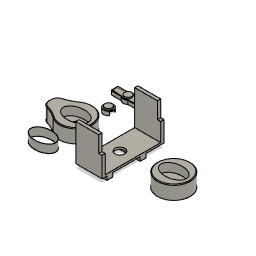
FPLock_Mach (Autodesk Fusion 360 design; units mm, degrees)
Autodesk Fusion 360 part; units mm, degrees
sketch "草图5" plane through (0, 0, 0) normal (0, 1, 0) x (1, 0, 0)
  line L0 (100, -50) -> (140, -50)
  line L1 (140, -50) -> (140, 45)
  line L2 (140, 45) -> (100, 45)
  line L3 (100, 45) -> (100, -50)
  constraint horizontal L0
  constraint vertical L1
  constraint horizontal L2
  constraint vertical L3
extrude "拉伸7" add sketch "草图5" along normal blind 3 makes body 1
sketch "草图6" plane through (0, 3, 0) normal (0, 1, 0) x (-1, 0, 0)
  line L0 (-100, -45) -> (-100, 50)
  line L1 (-100, 50) -> (-140, 50)
  line L2 (-140, 50) -> (-140, -45)
  line L3 (-140, -45) -> (-100, -45)
  line L4 (-100, -40) -> (-140, -40)
  line L5 (-140, -40) -> (-140, -45)
  line L6 (-140, -45) -> (-100, -45)
  line L7 (-100, -45) -> (-100, -40)
  line L8 (-140, 45) -> (-100, 45)
  line L9 (-100, 45) -> (-100, 50)
  line L10 (-100, 50) -> (-140, 50)
  line L11 (-140, 50) -> (-140, 45)
  constraint horizontal L4
  constraint vertical L5
  constraint horizontal L6
  constraint vertical L7
  constraint coincident L2.end L3.start
  constraint coincident L0 L4.start
  constraint horizontal L8
  constraint vertical L9
  constraint horizontal L10
  constraint vertical L11
  constraint coincident L0.end L1.start
  constraint coincident L2 L8.start
extrude "拉伸8" add sketch "草图6" along normal blind 47 contours L0 L2 L3 L4 L5 L6 L7 | L0 L1 L2 L8 L9 L10 L11 bodies 1
sketch "草图7" plane through (0, 3, 0) normal (0, 1, 0) x (-1, 0, 0)
  line L0 (-100, 45) -> (-140, 45)
  line L1 (-140, 45) -> (-140, -40)
  line L2 (-140, -40) -> (-100, -40)
  line L3 (-100, -40) -> (-100, 45)
  circle A0 centre (-120, 2.5) radius 7.5
  dimension "d80" = 15
  measures "d80" diameter of A0
extrude "拉伸9" cut sketch "草图7" against normal blind 3 contours A0 bodies 1
sketch "草图8" plane through (0, 0, -45) normal (0, 0, -1) x (-1, 0, 0)
  line L0 (-140, 0) -> (-100, 0)
  line L1 (-100, 0) -> (-100, 50)
  line L2 (-100, 50) -> (-140, 50)
  line L3 (-140, 50) -> (-140, 0)
sketch "草图11" plane through (0, 0, -45) normal (0, 0, -1) x (-1, 0, 0)
  line L0 (-135, 50) -> (-150, 50)
  line L1 (-150, 50) -> (-150, 25)
  line L2 (-150, 25) -> (-135, 25)
  line L3 (-135, 25) -> (-135, 50)
  constraint horizontal L0
  constraint vertical L1
  constraint horizontal L2
  constraint vertical L3
extrude "拉伸12" cut sketch "草图11" against normal blind 5 bodies 1
sketch "草图12" plane through (0, 0, 50) normal (0, 0, 1) x (1, 0, 0)
  line L0 (100, 0) -> (140, 0)
  line L1 (140, 0) -> (140, 50)
  line L2 (140, 50) -> (100, 50)
  line L3 (100, 50) -> (100, 0)
  line L4 (135, 25) -> (140, 25)
  line L5 (140, 25) -> (140, 50)
  line L6 (140, 50) -> (135, 50)
  line L7 (135, 50) -> (135, 25)
  constraint horizontal L4
  constraint vertical L5
  constraint horizontal L6
  constraint vertical L7
  constraint coincident L1.end L2.start
extrude "拉伸15" cut sketch "草图12" against normal blind 5 contours L1 L2 L4 L5 L6 L7 bodies 1
extrude "拉伸25" cut 2 faces at (138.3333, 25, -43.3333) (136.6667, 25, 48.3333) along direction (0, -1, 0) blind 1 on bodies 1 bodies 1
sketch "草图24" plane through (0, 0, 0) normal (0, -1, 0) x (1, 0, 0)
  circle A0 centre (120, 2.5) radius 7.5
  line L0 (100, 50) -> (100, -45)
  line L1 (100, -45) -> (140, -45)
  line L2 (140, -45) -> (140, 50)
  line L3 (140, 50) -> (100, 50)
  line L4 (140, 2.5) -> (100, 2.5)
  line L5 (120, 2.5) -> (120, -7.5)
  line L6 (120, -7.5) -> (120, 32.5)
  line L7 (120, 32.5) -> (120, 33.5)
  line L8 (120, 33.5) -> (140, 33.5)
  line L9 (140, 33.5) -> (100, 33.5)
  line L10 (100, 33.5) -> (100, 43.5)
  line L11 (100, 43.5) -> (140, 43.5)
  line L12 (140, 43.5) -> (140, 33.5)
  line L13 (120, -7.5) -> (120, -8.5)
  line L14 (120, -8.5) -> (140, -8.5)
  line L15 (140, -8.5) -> (100, -8.5)
  line L16 (100, -8.5) -> (100, -18.5)
  line L17 (100, -18.5) -> (140, -18.5)
  line L18 (140, -18.5) -> (140, -8.5)
  dimension "d82" = 10
  dimension "d83" = 10
  constraint midpoint L2 L4.start
  constraint midpoint L0 L4.end
  constraint coincident A0.centre L5.start
  constraint perpendicular L4 L5
  constraint parallel L0 L6
  constraint parallel L6 L7
  constraint coincident L2 L8.end
  constraint perpendicular L2 L8
  constraint horizontal L9
  constraint vertical L10
  constraint horizontal L11
  constraint vertical L12
  constraint parallel L6 L13
  constraint coincident L2 L14.end
  constraint perpendicular L2 L14
  constraint horizontal L15
  constraint vertical L16
  constraint horizontal L17
  constraint vertical L18
  measures "d82" distance of L8.end L11.end
  measures "d83" distance of L14.end L17.end
extrude "拉伸35" add sketch "草图24" along normal blind 6 contours L0 L2 L14 L15 L16 L17 L18 | L0 L2 L8 L9 L10 L11 L12 bodies 1
extrude "拉伸37" add 2 faces at (123.3333, 50, -41.6667) (123.3333, 50, 48.3333) along direction (0, 1, 0) blind 6 on bodies 1 bodies 1
extrude "拉伸38" add 2 faces at (138.3333, 24, -43.3333) (136.6667, 24, 48.3333) along direction (0, 1, 0) blind 7 on bodies 1 bodies 1
extrude "拉伸39" cut 1 faces at (113.3333, -2, -18.5) along direction (0, 0, 1) blind 1 on bodies 1 bodies 1
extrude "拉伸40" cut 1 faces at (113.3333, -2, 43.5) along direction (0, 0, -1) blind 1 on bodies 1 bodies 1
sketch "草图27" plane through (0, 0, 0) normal (0, 1, 0) x (1, 0, 0)
  circle A0 centre (200, 0) radius 25
extrude "拉伸41" add sketch "草图27" along normal blind 2 separate body makes body 2
sketch "草图28" plane through (0, 2, 0) normal (0, 1, 0) x (-1, 0, 0)
  circle A0 centre (-200, 0) radius 25
  ellipse E0 centre (-200, 0) end of major axis (-219, 0) minor radius 12.5
  line L0 (-181, 0) -> (-219, 0)
  line L1 (-200, 12.5) -> (-200, -12.5)
  ellipse E1 centre (-200, 0) end of major axis (-200, -13) minor radius 19.5
  line L2 (-200, 13) -> (-200, -13)
  line L3 (-219.5, 0) -> (-180.5, 0)
  dimension "d100" = 25
  constraint concentric A0 E0
  constraint horizontal L0
  constraint coincident E0 L0.start
  constraint coincident E0 L0.end
  constraint coincident E0 L1.start
  constraint coincident E0 L1.end
  constraint concentric E0 E1
  constraint perpendicular L0 L2
  constraint coincident E1 L2.start
  constraint coincident E1 L2.end
  constraint coincident E1 L3.start
  constraint coincident E1 L3.end
extrude "拉伸44" add sketch "草图28" along normal blind 13 bodies 2
fillet "圆角8" radius 1 1 edges at (223.3082, 15, -9.0404) on bodies 2
sketch "草图29" plane through (0, 0, 0) normal (0, -1, 0) x (1, 0, 0)
  circle A0 centre (200, 0) radius 25
  circle A1 centre (200, 0) radius 20
  line L0 (220, 6.5) -> (180, 6.5)
  line L1 (180, 6.5) -> (180, -6.5)
  line L2 (180, -6.5) -> (220, -6.5)
  line L3 (220, -6.5) -> (220, 6.5)
  constraint concentric A0 A1
  constraint horizontal L0
  constraint vertical L1
  constraint horizontal L2
  constraint vertical L3
extrude "拉伸45" add sketch "草图29" along normal blind 6 contours A0 | A1 L0 | A1 L2 bodies 2
sketch "草图30" plane through (0, 0, 0) normal (0, -1, 0) x (1, 0, 0)
  line L0 (220, 6.5) -> (180, 6.5)
  line L1 (180, 6.5) -> (180, -6.5)
  line L2 (180, -6.5) -> (220, -6.5)
  line L3 (220, -6.5) -> (220, 6.5)
  circle A0 centre (200, 0) radius 2.5
extrude "拉伸46" cut sketch "草图30" against normal blind 2 contours A0 bodies 2
fillet "圆角9" radius 1 1 edges at (197.6692, 2, -0.904) on bodies 2
sketch "草图31" plane through (0, 0, 0) normal (0, -1, 0) x (1, 0, 0)
  circle A0 centre (200, 0) radius 2.5
  line L0 (220, 6.5) -> (180, 6.5)
  line L1 (180, 6.5) -> (180, -6.5)
  line L2 (180, -6.5) -> (220, -6.5)
  line L3 (220, -6.5) -> (220, 6.5)
  line L4 (206, 6.5) -> (220, 3)
  line L5 (220, -3) -> (206, -6.5)
  line L6 (200, 13) -> (200, -13)
  line L7 (194, 6.5) -> (180, 3)
  line L8 (180, -3) -> (194, -6.5)
  constraint coincident L0 L4.start
  constraint coincident L3 L4.end
  constraint coincident L3 L5.start
  constraint coincident L2 L5.end
  constraint perpendicular L2 L6
  constraint symmetric L4.start L6 L7.start
  constraint symmetric L4.end L6 L7.end
  constraint symmetric L5.start L6 L8.start
  constraint symmetric L5.end L6 L8.end
extrude "拉伸47" add sketch "草图31" along normal blind 6 contours L0 L3 L4 | L0 L1 L7 | L1 L2 L8 | L2 L3 L5 bodies 2
sketch "草图32" plane through (0, 0, 0) normal (0, 1, 0) x (1, 0, 0)
  circle A0 centre (50, 0) radius 25
extrude "拉伸48" add sketch "草图32" along normal blind 2 separate body makes body 3
sketch "草图33" plane through (0, 2, 0) normal (0, 1, 0) x (-1, 0, 0)
  circle A0 centre (-50, 0) radius 25
  ellipse E0 centre (-50, 0) end of major axis (-69, 0) minor radius 12.5
  line L0 (-31, 0) -> (-69, 0)
  line L1 (-50, 12.5) -> (-50, -12.5)
  ellipse E1 centre (-50, 0) end of major axis (-69.5, 0) minor radius 13
  line L2 (-30.5, 0) -> (-69.5, 0)
  line L3 (-50, 13) -> (-50, -13)
  dimension "d121" = 25
  constraint concentric A0 E0
  constraint horizontal L0
  constraint coincident E0 L0.start
  constraint coincident E0 L0.end
  constraint coincident E0 L1.start
  constraint coincident E0 L1.end
  constraint concentric E0 E1
  constraint perpendicular L1 L2
  constraint coincident E1 L2.start
  constraint coincident E1 L2.end
  constraint coincident E1 L3.start
  constraint coincident E1 L3.end
extrude "拉伸49" add sketch "草图33" along normal blind 13 bodies 3
sketch "草图34" plane through (0, 0, 0) normal (0, -1, 0) x (1, 0, 0)
  circle A0 centre (50, 0) radius 25
  circle A1 centre (50, 0) radius 22
  circle A2 centre (50, 0) radius 6
  line L0 (57, 4.5) -> (57, -4.5)
  line L1 (43, 4.5) -> (43, -4.5)
  line L2 (57, 4.5) -> (71.5349, 4.5)
  line L3 (57, 4.5) -> (57, 20.8567)
  line L4 (43, -4.5) -> (28.4651, -4.5)
  line L5 (43, -4.5) -> (43, -20.8567)
  constraint concentric A0 A1
  constraint concentric A1 A2
  constraint vertical L0
  constraint parallel L0 L1
  constraint coincident A1 L2.end
  constraint perpendicular L0 L2
  constraint coincident A1 L3.end
  constraint perpendicular L2 L3
  constraint coincident A1 L4.end
  constraint perpendicular L1 L4
  constraint coincident A1 L5.end
  constraint perpendicular L4 L5
extrude "拉伸50" add sketch "草图34" along normal blind 6 contours A0 | A1 L2 L3 | A1 L4 L5 bodies 3
extrude "拉伸51" cut sketch "草图34" against normal blind 2 contours A2 bodies 3
sketch "草图35" plane through (0, -6, 0) normal (0, -1, 0) x (1, 0, 0)
  line L0 (57, 20.8567) -> (57, 4.5)
  line L1 (57, 4.5) -> (71.5349, 4.5)
  arc A0 (43, -20.8567) -> (71.5349, 4.5) centre (50, 0) ccw
  line L2 (43, -20.8567) -> (43, -4.5)
  line L3 (43, -4.5) -> (28.4651, -4.5)
  arc A1 (57, 20.8567) -> (28.4651, -4.5) centre (50, 0) ccw
  circle A2 centre (50, 0) radius 25
  line L4 (57, 5.5) -> (71.5349, 4.5)
  line L5 (43, -5.5) -> (28.4651, -4.5)
  constraint coincident L0 L4.start
  constraint coincident L1.end A0.end
  constraint coincident L2 L5.start
  constraint coincident L3.end A1.end
extrude "拉伸52" cut sketch "草图35" against normal blind 6 contours L0 L1 L4 | L2 L3 L5 bodies 3
sketch "草图36" plane through (0, 0, 0) normal (0, 1, 0) x (1, 0, 0)
  ellipse E0 centre (50, -50) end of major axis (69.25, -50) minor radius 12.75
  line L0 (30.75, -50) -> (69.25, -50)
  line L1 (50, -62.75) -> (50, -37.25)
  ellipse E1 centre (50, -50) end of major axis (69, -50) minor radius 12.5
  line L2 (31, -50) -> (69, -50)
  line L3 (50, -62.5) -> (50, -37.5)
  constraint horizontal L0
  constraint coincident E0 L0.start
  constraint coincident E0 L0.end
  constraint coincident E0 L1.start
  constraint coincident E0 L1.end
  constraint concentric E0 E1
  constraint perpendicular L1 L2
  constraint coincident E1 L2.start
  constraint coincident E1 L2.end
  constraint coincident E1 L3.start
  constraint coincident E1 L3.end
extrude "拉伸53" add sketch "草图36" along normal blind 12.5 separate body contours E0 L0 L1 E1 | E0 L0 L1 E1 | E0 L0 L1 E1 | E0 L0 L1 E1 makes body 4
sketch "草图37" plane through (0, 0, 0) normal (0, 1, 0) x (1, 0, 0)
  circle A0 centre (50, 50) radius 5.5
extrude "拉伸54" add sketch "草图37" along normal blind 2 separate body makes body 5
sketch "草图38" plane through (0, 0, 0) normal (0, -1, 0) x (1, 0, 0)
  circle A0 centre (50, -50) radius 5.5
  circle A1 centre (50, -50) radius 7.5
  dimension "d136" = 15
  constraint concentric A0 A1
  measures "d136" diameter of A1
extrude "拉伸55" add sketch "草图38" along normal blind 1 contours A0 | A1 bodies 5
sketch "草图39" plane through (0, -1, 0) normal (0, -1, 0) x (1, 0, 0)
  circle A0 centre (50, -50) radius 7.5
  circle A1 centre (50, -50) radius 6.25
  line L0 (42.5, -45.5) -> (57.5, -45.5)
  line L1 (57.5, -45.5) -> (57.5, -54.5)
  line L2 (57.5, -54.5) -> (42.5, -54.5)
  line L3 (42.5, -54.5) -> (42.5, -45.5)
  dimension "d139" = 12.5
  constraint concentric A0 A1
  constraint horizontal L0
  constraint vertical L1
  constraint horizontal L2
  constraint vertical L3
  measures "d139" diameter of A1
extrude "拉伸56" add sketch "草图39" along normal blind 5 contours A0 A1 L0 | A0 A1 L2 bodies 5
sketch "草图42" plane through (0, -6, 0) normal (0, -1, 0) x (1, 0, 0)
  circle A0 centre (50, 0) radius 25
  line L0 (57, 5.5) -> (71.5349, 4.5)
  arc A1 (43, -20.8567) -> (71.5349, 4.5) centre (50, 0) ccw
  line L1 (43, -20.8567) -> (43, -5.5)
  line L2 (43, -5.5) -> (28.4651, -4.5)
  arc A2 (57, 20.8567) -> (28.4651, -4.5) centre (50, 0) ccw
  line L3 (57, 20.8567) -> (57, 5.5)
  line L4 (95, 0) -> (0, 0)
  arc A3 (50, -35) -> (10, -10) centre (0.7557, -69.2908) ccw
  line L5 (10, -10) -> (10, 10)
  arc A4 (10, 10) -> (50, 35) centre (0.7557, 69.2908) ccw
  constraint coincident L4.end origin
  constraint horizontal L4
extrude "拉伸60" add sketch "草图42" against normal blind 21 contours A0 L4 L5 A4 | A0 L4 A3 L5 bodies 3
fillet "圆角13" radius 10 2 edges at (10, 4.5, 10) (10, 4.5, -10) on bodies 3
fillet "圆角14" radius 1 6 edges at (26.7579, 15, -15.2099) (12.016, 15, -8.0019) (10, 15, 0) (12.016, 15, 8.0019) (26.7578, 15, 15.2099) (75, 15, 0.0001) on bodies 3
fillet "圆角15" radius 2 2 edges at (57, -3, 5.5) (43, -3, -5.5) on bodies 3
copy_body "复制和粘贴实体3" bodies 5 makes body 6
move_body "移动7" bodies 6 to x (1, 0, 0) y (0, 1, 0) z (0, 0, 1) at (0, 0, -30)
sketch "草图43" plane through (0, -1, 0) normal (0, -1, 0) x (1, 0, 0)
  line L0 (54.3373, -84.5) -> (56, -84.5)
  arc A0 (56, -84.5) -> (56, -75.5) centre (50, -80) ccw
  line L1 (56, -75.5) -> (54.3373, -75.5)
  arc A1 (54.3373, -75.5) -> (45.6627, -75.5) centre (50, -80) ccw
  line L2 (45.6627, -75.5) -> (44, -75.5)
  arc A2 (44, -75.5) -> (44, -84.5) centre (50, -80) ccw
  line L3 (44, -84.5) -> (45.6627, -84.5)
  arc A3 (45.6627, -84.5) -> (54.3373, -84.5) centre (50, -80) ccw
  line L4 (29, -74.5) -> (45, -74.5)
  line L5 (45, -74.5) -> (45, -85.5)
  line L6 (45, -85.5) -> (29, -85.5)
  line L7 (29, -85.5) -> (29, -74.5)
  line L8 (50, -70) -> (50, -90)
  line L9 (71, -74.5) -> (55, -74.5)
  line L10 (71, -85.5) -> (71, -74.5)
  line L11 (55, -74.5) -> (55, -85.5)
  line L12 (55, -85.5) -> (71, -85.5)
  constraint horizontal L4
  constraint vertical L5
  constraint horizontal L6
  constraint vertical L7
  constraint vertical L8
  constraint symmetric L4.start L8 L9.start
  constraint symmetric L4.end L8 L9.end
  constraint symmetric L5.end L8 L11.end
  constraint symmetric L6.end L8 L10.start
extrude "拉伸61" add sketch "草图43" against normal blind 1 contours L0 A0 L1 L9 L10 L11 L12 | L2 A2 L3 L4 L5 L6 L7 bodies 6
sketch "草图44" plane through (0, -1, 0) normal (0, -1, 0) x (1, 0, 0)
  line L0 (54.3373, -84.5) -> (56, -84.5)
  arc A0 (55.099, -85.5) -> (56, -84.5) centre (50, -80) ccw
  line L1 (55.099, -85.5) -> (71, -85.5)
  line L2 (71, -85.5) -> (71, -74.5)
  line L3 (71, -74.5) -> (55.099, -74.5)
  arc A1 (56, -75.5) -> (55.099, -74.5) centre (50, -80) ccw
  line L4 (56, -75.5) -> (54.3373, -75.5)
  arc A2 (54.3373, -75.5) -> (45.6627, -75.5) centre (50, -80) ccw
  line L5 (45.6627, -75.5) -> (44, -75.5)
  arc A3 (44.901, -74.5) -> (44, -75.5) centre (50, -80) ccw
  line L6 (44.901, -74.5) -> (29, -74.5)
  line L7 (29, -74.5) -> (29, -85.5)
  line L8 (29, -85.5) -> (44.901, -85.5)
  arc A4 (44, -84.5) -> (44.901, -85.5) centre (50, -80) ccw
  line L9 (44, -84.5) -> (45.6627, -84.5)
  arc A5 (45.6627, -84.5) -> (54.3373, -84.5) centre (50, -80) ccw
  line L10 (30, -75.5) -> (70, -75.5)
  line L11 (70, -75.5) -> (70, -84.5)
  line L12 (70, -84.5) -> (30, -84.5)
  line L13 (30, -84.5) -> (30, -75.5)
  line L14 (25, -80) -> (75, -80)
  line L15 (50, -70) -> (50, -90)
  line L16 (30, -77) -> (45.6627, -75.5)
  line L17 (70, -77) -> (54.3373, -75.5)
  line L18 (70, -83) -> (54.3373, -84.5)
  line L19 (30, -83) -> (45.6627, -84.5)
  constraint horizontal L10
  constraint vertical L11
  constraint horizontal L12
  constraint vertical L13
  constraint perpendicular L2 L14
  constraint perpendicular L14 L15
  constraint coincident L13 L16.start
  constraint coincident A2.end L5.start
  constraint symmetric L15 L16.start L17.start
  constraint symmetric L15 A2.end L4.end
  constraint symmetric L14 L16.start L19.start
  constraint symmetric L14 A2.end L9.end
  constraint symmetric L14 L17.start L18.start
  constraint symmetric L14 L4.end L0.start
extrude "拉伸62" add sketch "草图44" along normal blind 5 contours L0 L11 L12 L18 | A0 L1 L2 L11 L12 L14 | L9 L12 L13 L19 | L2 L3 A1 L10 L11 L14 | L7 L8 A4 L12 L13 L14 | A3 L6 L7 L10 L13 L14 | L4 L10 L11 L17 | L5 L10 L13 L16 bodies 6
fillet "圆角16" radius 1 4 edges at (45.6627, -3.5, -84.5) (54.3373, -3.5, -84.5) (54.3373, -3.5, -75.5) (45.6627, -3.5, -75.5) on bodies 6
fillet "圆角17" radius 1 4 edges at (71, -3, -85.5) (71, -3, -74.5) (29, -3, -85.5) (29, -3, -74.5) on bodies 6
fillet "圆角18" radius 0.5 12 edges at (50, 0, -87.5) (37.4505, 0, -85.5) (29.2929, 0, -85.2071) (29, 0, -80) (29.2929, 0, -74.7929) (37.4505, 0, -74.5) (50, 0, -72.5) (62.5495, 0, -74.5) (70.7071, 0, -74.7929) (71, 0, -80) (70.7071, 0, -85.2071) (62.5495, 0, -85.5) on bodies 6
sketch "草图45" plane through (0, -1, 0) normal (0, -1, 0) x (1, 0, 0)
  line L0 (70, -77) -> (54.6704, -75.5319)
  arc A0 (54.1084, -75.29) -> (54.6704, -75.5319) centre (54.7657, -74.5365) ccw
  arc A1 (54.1084, -75.29) -> (45.8916, -75.29) centre (50, -80) ccw
  arc A2 (45.3296, -75.5319) -> (45.8916, -75.29) centre (45.2343, -74.5365) ccw
  line L1 (45.3296, -75.5319) -> (30, -77)
  line L2 (30, -77) -> (30, -83)
  line L3 (30, -83) -> (45.3296, -84.4681)
  arc A3 (45.8916, -84.71) -> (45.3296, -84.4681) centre (45.2343, -85.4636) ccw
  arc A4 (45.8916, -84.71) -> (54.1084, -84.71) centre (50, -80) ccw
  arc A5 (54.6704, -84.4681) -> (54.1084, -84.71) centre (54.7657, -85.4636) ccw
  line L4 (54.6704, -84.4681) -> (70, -83)
  line L5 (70, -83) -> (70, -77)
  circle A6 centre (50, -80) radius 3
  dimension "d170" = 6
  constraint concentric A1 A6
  measures "d170" diameter of A6
extrude "拉伸63" cut sketch "草图45" against normal blind 1 contours A6 bodies 6
